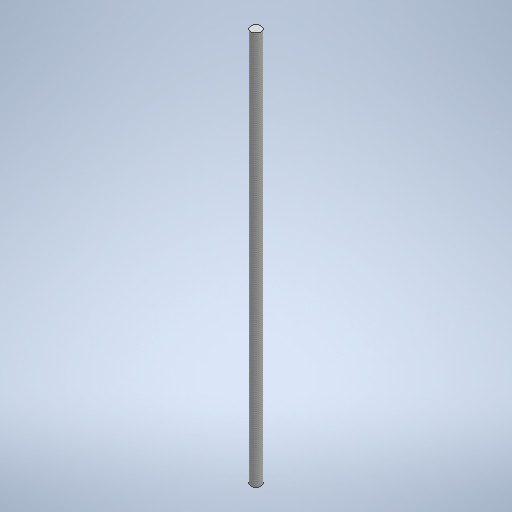
# Autodesk Inventor part: tornillo
Saved by Autodesk Inventor 2025.2 (Build 292293000, 293)
## iProperties
Created: 2025-11-05
Part Number: tornillo
Material: Genérico
Document SubType Name: Modeling
Designer: Jonathan Galarza
Density: 1 g/cm^3
Appearance: Valor por defecto
Author: Jonathan Galarza
Autodesk Inventor part; units mm, degrees
ref_plane "YZ Plane" through (0, 0, 0) normal (1, 0, 0) x (0, 1, 0)
ref_plane "XZ Plane" through (0, 0, 0) normal (0, 1, 0) x (-1, 0, 0)
ref_plane "XY Plane" through (0, 0, 0) normal (0, 0, 1) x (1, 0, 0)
sketch "Boceto1" plane through (0, 0, 0) normal (0, 1, 0) x (-1, 0, 0)
  circle A0 centre (0, 0) radius 4
  dimension "d0" = 8
  constraints: 1 centre point, 1 coincident
  measures "d0" diameter of A0
extrude "Extrusión1" add sketch "Boceto1" along normal blind 400
thread "Rosca1" size "M8x1.25" class "6g" standard "ISO Metric profile" full length
sketch "Boceto2" plane through (0, 400, 0) normal (0, 1, 0) x (1, 0, 0)
  circle A0 centre (0, 0) radius 4
  constraints: 1 centre point, 1 coincident
extrude "Extrusión2" cut sketch "Boceto2" against normal blind 23
sketch "Boceto3" plane through (0, 377, 0) normal (0, 1, 0) x (1, 0, 0)
  circle A0 centre (0, 0) radius 4
  constraints: 1 centre point, 1 coincident
extrude "Extrusión3" cut sketch "Boceto3" against normal blind 77
